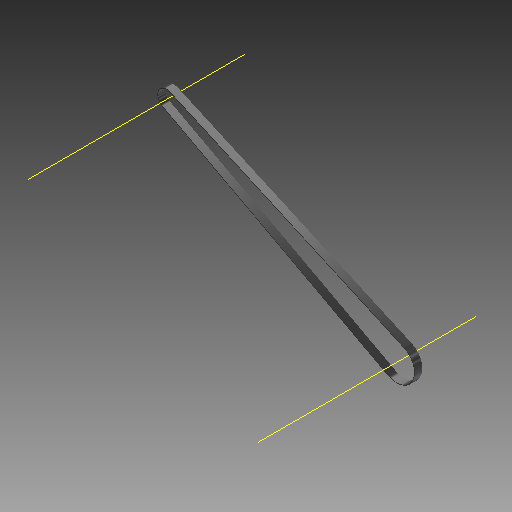
# Autodesk Inventor part: Synchronous Belt
Saved by Autodesk Inventor 2019.4 (Build 234330000, 330)
## iProperties
Created: 2020-02-16
Part Number: Synchronous Belt
Material: Rubber
Document SubType Name: Modeling
Designer: admin
Density: 0.93 g/cm^3
Appearance: Rubber - Black - Version 1.1
Mass: 7.44001 g
Surface Area: 176 cm^2
Volume: 8.00001 cm^3
CustomPartVersion: 1
Author: admin
Autodesk Inventor part; units mm, degrees
sketch "Sketch Path" plane through (0, 0, 0) normal (0, 0, 1) x (1, 0, 0)
  arc A0 (147.4989, -88.898) -> (168.4685, -46.0349) centre (158.7288, -67.831) ccw
  arc A1 (-144.9943, 94.0378) -> (-155.4791, 72.6063) centre (-149.8642, 83.1398) ccw
  line L0 (-144.9943, 94.0378) -> (168.4685, -46.0349)
  line L1 (147.4989, -88.898) -> (-155.4791, 72.6063)
  constraints: 4 end point, 4 point on circle, 2 centre point
ref_plane "Cross Section Plane" through (168.4685, -46.0349, 0) normal (-0.913, 0.408, 0) x (0, 0, 1)
ref_plane "Work Plane2" through (158.7288, -67.831, 0) normal (-1, 0, 0) x (0, 0, 1)
ref_plane "Work Plane3" through (-149.8642, 83.1398, 0) normal (0.6166, -0.7872, 0) x (0, 0, 1)
sketch "Cross Section" plane through (168.4685, -46.0349, 0) normal (-0.913, 0.408, 0) x (0, 0, 1)
  line L0 (-5, 0.5) -> (5, 0.5)
  line L1 (5, 0.5) -> (5, -0.5)
  line L2 (5, -0.5) -> (-5, -0.5)
  line L3 (-5, -0.5) -> (-5, 0.5)
  line L4 (-5, 0) -> (5, 0) construction
  point P0 (0, 0)
  point P1 (0, 0)
  dimension "d0" = 10
  dimension "d4" = 0.5
  dimension "d5" = 0.5
  constraints: 10 end point, 3 midpoint, 2 parallel, 1 coincident, 1 horizontal, 1 perpendicular, 1 other
  measures "d0" distance between parallel lines of L1 L3
  measures "d4" distance between parallel lines of L2 L4
  measures "d5" distance between parallel lines of L4 L0
sweep "Belt" add profiles "Cross Section" path "Sketch Path"
equation "\"d0\" = da_B"
equation "\"d4\" = da_a"
equation "\"d5\" = da_a2"
equation "\"da_B\" = 10"
equation "\"da_pb\" = 5"
equation "\"da_L\" = 800.00079"
equation "\"da_a\" = 0.5"
equation "\"da_S\" = 2.65"
equation "\"da_Beta\" = 20deg"
equation "\"da_Ht\" = 1.2"
equation "\"da_H\" = 2.2"
equation "\"da_a2\" = 0.5"
body "Solid1"
